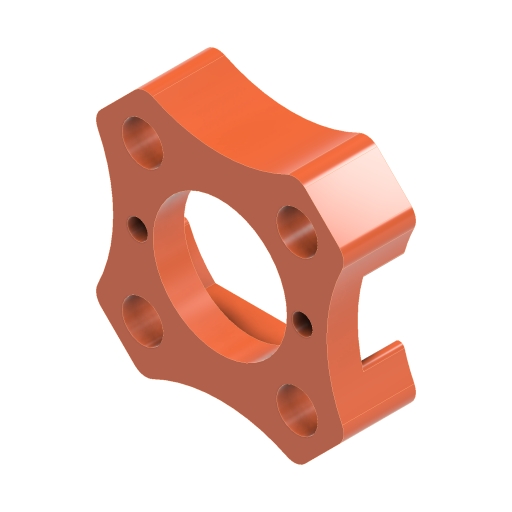
# Autodesk Inventor part: WobbleX WS12 Bottom
Saved by Autodesk Inventor 2023.2 (Build 272271000, 271)
## iProperties
Created: 2023-02-17
Part Number: WobbleX WS12 Bottom
Material: ABS Plastic
Document SubType Name: Modeling
Designer: remop
Density: 1.06 g/cm^3
Appearance: Smooth - Light Orange
Author: remop
Autodesk Inventor part; units mm, degrees
ref_plane "YZ Plane" through (0, 0, 0) normal (1, 0, 0) x (0, 1, 0)
ref_plane "XZ Plane" through (0, 0, 0) normal (0, 1, 0) x (-1, 0, 0)
ref_plane "XY Plane" through (0, 0, 0) normal (0, 0, 1) x (1, 0, 0)
sketch "Sketch1" plane through (0, 0, 0) normal (0, 0, 1) x (1, 0, 0)
  arc A0 (16.5324, 32.4843) -> (13.101, 33.0618) centre (14.4111, 30.3629) ccw projected
  arc A1 (-13.101, 33.0618) -> (13.101, 33.0618) centre (0, 60.05) ccw projected
  arc A2 (-13.101, 33.0618) -> (-16.5324, 32.4843) centre (-14.4111, 30.3629) ccw projected
  line L0 (-23.1843, 25.8324) -> (-16.5324, 32.4843) projected
  arc A3 (-23.1843, 25.8324) -> (-23.7618, 22.401) centre (-21.0629, 23.7111) ccw projected
  arc A4 (-23.7618, -3.801) -> (-23.7618, 22.401) centre (-50.75, 9.3) ccw projected
  arc A5 (-23.7618, -3.801) -> (-23.1843, -7.2324) centre (-21.0629, -5.1111) ccw projected
  line L1 (-16.5324, -13.8843) -> (-23.1843, -7.2324) projected
  arc A6 (-16.5324, -13.8843) -> (-13.101, -14.4618) centre (-14.4111, -11.7629) ccw projected
  arc A7 (13.101, -14.4618) -> (-13.101, -14.4618) centre (0, -41.45) ccw projected
  arc A8 (13.101, -14.4618) -> (16.5324, -13.8843) centre (14.4111, -11.7629) ccw projected
  line L2 (23.1843, -7.2324) -> (16.5324, -13.8843) projected
  arc A9 (23.1843, -7.2324) -> (23.7618, -3.801) centre (21.0629, -5.1111) ccw projected
  arc A10 (23.7618, 22.401) -> (23.7618, -3.801) centre (50.75, 9.3) ccw projected
  arc A11 (23.7618, 22.401) -> (23.1843, 25.8324) centre (21.0629, 23.7111) ccw projected
  line L3 (16.5324, 32.4843) -> (23.1843, 25.8324) projected
  circle A12 centre (15, 24.3) radius 4 projected
  circle A13 centre (15, -5.7) radius 4 projected
  circle A14 centre (-15, -5.7) radius 4 projected
  circle A15 centre (-15, 24.3) radius 4 projected
  circle A16 centre (0, 9.3) radius 13 projected
  circle A17 centre (-16, 9.3) radius 2
  circle A18 centre (16, 9.3) radius 2
  point P0 (0, 0)
  dimension "d6" = 32
  dimension "d7" = 4
  dimension "d8" = 16
  constraints: 2 centre point, 2 horizontal alignment, 1 equal radius
  measures "d6" distance of A18.centre A17.centre
  measures "d7" diameter of A17
  measures "d8" distance of A16.centre A17.centre
extrude "Extrusion1" add sketch "Sketch1" along normal blind 6
sketch "Sketch2" plane through (0, 0, 0) normal (0, 0, -1) x (-1, 0, 0)
  line L0 (14.6969, -5.7) -> (-14.6969, -5.7) projected
  arc A0 (14.6969, -5.7) -> (14.6969, 24.3) centre (0, 9.3) ccw projected
  line L1 (-14.6969, 24.3) -> (14.6969, 24.3) projected
  arc A1 (-14.6969, 24.3) -> (-14.6969, -5.7) centre (0, 9.3) ccw projected
  circle A2 centre (0, 9.3) radius 6 projected
  circle A3 centre (-11.3137, -2.0137) radius 2.4 projected
  circle A4 centre (11.3137, -2.0137) radius 2.4 projected
  circle A5 centre (16, 9.3) radius 2.4 projected
  circle A6 centre (11.3137, 20.6137) radius 2.4 projected
  circle A7 centre (-11.3137, 20.6137) radius 2.4 projected
  circle A8 centre (-16, 9.3) radius 2.4 projected
  arc A9 (14.8997, -6.2) -> (14.8997, 24.8) centre (0, 9.3) ccw
  line L2 (14.8997, -6.2) -> (-14.8997, -6.2)
  arc A10 (-14.8997, 24.8) -> (-14.8997, -6.2) centre (0, 9.3) ccw
  line L3 (-14.8997, 24.8) -> (14.8997, 24.8)
  line L4 (-23.1843, 25.8324) -> (-16.5324, 32.4843) projected
  arc A11 (-23.1843, 25.8324) -> (-23.7618, 22.401) centre (-21.0629, 23.7111) ccw projected
  arc A12 (-23.7618, -3.801) -> (-23.7618, 22.401) centre (-50.75, 9.3) ccw projected
  arc A13 (-23.7618, -3.801) -> (-23.1843, -7.2324) centre (-21.0629, -5.1111) ccw projected
  line L5 (-16.5324, -13.8843) -> (-23.1843, -7.2324) projected
  arc A14 (-16.5324, -13.8843) -> (-13.101, -14.4618) centre (-14.4111, -11.7629) ccw projected
  arc A15 (13.101, -14.4618) -> (-13.101, -14.4618) centre (0, -41.45) ccw projected
  arc A16 (13.101, -14.4618) -> (16.5324, -13.8843) centre (14.4111, -11.7629) ccw projected
  line L6 (23.1843, -7.2324) -> (16.5324, -13.8843) projected
  arc A17 (23.1843, -7.2324) -> (23.7618, -3.801) centre (21.0629, -5.1111) ccw projected
  arc A18 (23.7618, 22.401) -> (23.7618, -3.801) centre (50.75, 9.3) ccw projected
  arc A19 (23.7618, 22.401) -> (23.1843, 25.8324) centre (21.0629, 23.7111) ccw projected
  line L7 (16.5324, 32.4843) -> (23.1843, 25.8324) projected
  arc A20 (16.5324, 32.4843) -> (13.101, 33.0618) centre (14.4111, 30.3629) ccw projected
  arc A21 (-13.101, 33.0618) -> (13.101, 33.0618) centre (0, 60.05) ccw projected
  arc A22 (-13.101, 33.0618) -> (-16.5324, 32.4843) centre (-14.4111, 30.3629) ccw projected
  circle A23 centre (-15, -5.7) radius 4 projected
  circle A24 centre (15, -5.7) radius 4 projected
  circle A25 centre (15, 24.3) radius 4 projected
  circle A26 centre (-15, 24.3) radius 4 projected
  circle A27 centre (0, 9.3) radius 13 projected
  point P0 (0, 0)
  point P1 (21.0622, 4.9833)
  point P2 (-21.0622, 4.9833)
  point P3 (-21.0622, 13.6167)
  point P4 (21.0622, 13.6167)
  dimension "d2" = 0.5
  constraints: 4 end point, 4 point on circle, 2 centre point, 3 other
  measures "d2" distance between parallel lines of L1 L3
extrude "Extrusion2" add sketch "Sketch2" along normal blind 8 contours A23 A10 L2 | L2 A24 A9 A18 A17 L6 A16 A15 A14 L5 A13 A12 A10 A23 | L2 A9 A24 | A12 A11 L4 A22 A21 A20 L7 A19 A18 A9 A25 L3 A26 A10 | A26 L3 A10 | A9 L3 A25
fillet "Fillet1" radius 1 4 edges at (-21.0622, 13.6167, -4) (-21.0622, 4.9833, -4) (21.0622, 4.9833, -4) (21.0622, 13.6167, -4)
equation "\"d8\" = 0.5 * d6"
body "Solid1"
